PTFE Box Test_v2 (Autodesk Fusion 360 design; units mm, degrees)
Autodesk Fusion 360 part; units mm, degrees
box "BoxPrimitive1" add length 203.2 width 203.2 height 5.08 placed x (0, 0, -1) y (-1, 0, 0) z (0, 1, 0) at (203.2, 0, 0)
hole "Hole1" at (101.6, 5.08, -101.6) direction (0, -1, 0) diameter 101.6 depth 2 tip angle 180
